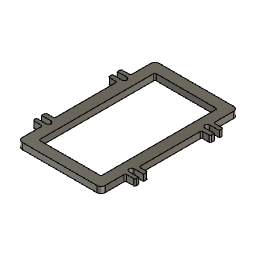
Model 2 v1 (Autodesk Fusion 360 design; units mm, degrees)
Autodesk Fusion 360 part; units mm, degrees
sketch "Sketch1" plane through (0, 0, 0) normal (0, 0, 1) x (1, 0, 0)
  line L0 (242.5602, 1007.653) -> (332.5602, 1007.653)
  line L1 (232.5602, 997.653) -> (232.5602, 952)
  line L2 (229.5602, 949) -> (212.5602, 949)
  line L3 (209.5602, 946) -> (209.5602, 940)
  line L4 (209.5602, 940) -> (229.5602, 940)
  arc A0 (242.5602, 1007.653) -> (232.5602, 997.653) centre (242.5602, 997.653) ccw
  line L5 (260.5602, 982.653) -> (332.5602, 982.653)
  line L6 (229.5602, 928) -> (209.5602, 928)
  line L7 (209.5602, 928) -> (209.5602, 921.1082)
  line L8 (212.5602, 918.1082) -> (227.6643, 918.1082)
  line L9 (229.5602, 940) -> (232.5602, 940)
  line L10 (229.5602, 928) -> (232.5602, 928)
  arc A1 (232.5602, 928) -> (232.5602, 940) centre (232.5602, 934) ccw
  line L11 (230.6643, 915.1082) -> (230.6643, 842.653)
  line L12 (257.5602, 979.653) -> (257.5602, 842.653)
  arc A2 (229.5602, 949) -> (232.5602, 952) centre (229.5602, 952) ccw
  arc A3 (230.6643, 915.1082) -> (227.6643, 918.1082) centre (227.6643, 915.1082) ccw
  arc A4 (212.5602, 949) -> (209.5602, 946) centre (212.5602, 946) ccw
  arc A5 (209.5602, 921.1082) -> (212.5602, 918.1082) centre (212.5602, 921.1082) ccw
  line L13 (435.5602, 949) -> (452.5602, 949)
  arc A6 (432.5602, 940) -> (432.5602, 928) centre (432.5602, 934) ccw
  line L14 (435.5602, 928) -> (432.5602, 928)
  line L15 (407.5602, 979.653) -> (407.5602, 842.653)
  line L16 (434.4561, 915.1082) -> (434.4561, 842.653)
  arc A7 (432.5602, 952) -> (435.5602, 949) centre (435.5602, 952) ccw
  line L17 (452.5602, 918.1082) -> (437.4561, 918.1082)
  arc A8 (432.5602, 997.653) -> (422.5602, 1007.653) centre (422.5602, 997.653) ccw
  line L18 (435.5602, 940) -> (432.5602, 940)
  arc A9 (437.4561, 918.1082) -> (434.4561, 915.1082) centre (437.4561, 915.1082) ccw
  arc A10 (452.5602, 918.1082) -> (455.5602, 921.1082) centre (452.5602, 921.1082) ccw
  line L19 (455.5602, 940) -> (435.5602, 940)
  line L20 (455.5602, 946) -> (455.5602, 940)
  line L21 (455.5602, 928) -> (455.5602, 921.1082)
  line L22 (422.5602, 1007.653) -> (332.5602, 1007.653)
  line L23 (404.5602, 982.653) -> (332.5602, 982.653)
  line L24 (432.5602, 997.653) -> (432.5602, 952)
  line L25 (435.5602, 928) -> (455.5602, 928)
  arc A11 (455.5602, 946) -> (452.5602, 949) centre (452.5602, 946) ccw
  line L26 (435.5602, 757.3059) -> (432.5602, 757.3059)
  line L27 (232.5602, 687.653) -> (232.5602, 733.3059)
  arc A12 (227.6643, 767.1978) -> (230.6643, 770.1978) centre (227.6643, 770.1978) ccw
  arc A13 (435.5602, 736.3059) -> (432.5602, 733.3059) centre (435.5602, 733.3059) ccw
  line L28 (212.5602, 767.1978) -> (227.6643, 767.1978)
  line L29 (455.5602, 757.3059) -> (455.5602, 764.1978)
  line L30 (229.5602, 757.3059) -> (232.5602, 757.3059)
  line L31 (435.5602, 736.3059) -> (452.5602, 736.3059)
  arc A14 (422.5602, 677.653) -> (432.5602, 687.653) centre (422.5602, 687.653) ccw
  line L32 (209.5602, 745.3059) -> (229.5602, 745.3059)
  arc A15 (209.5602, 739.3059) -> (212.5602, 736.3059) centre (212.5602, 739.3059) ccw
  arc A16 (232.5602, 733.3059) -> (229.5602, 736.3059) centre (229.5602, 733.3059) ccw
  arc A17 (232.5602, 687.653) -> (242.5602, 677.653) centre (242.5602, 687.653) ccw
  line L33 (455.5602, 739.3059) -> (455.5602, 745.3059)
  arc A18 (455.5602, 764.1978) -> (452.5602, 767.1978) centre (452.5602, 764.1978) ccw
  line L34 (209.5602, 757.3059) -> (209.5602, 764.1978)
  line L35 (229.5602, 745.3059) -> (232.5602, 745.3059)
  line L36 (209.5602, 739.3059) -> (209.5602, 745.3059)
  arc A19 (432.5602, 757.3059) -> (432.5602, 745.3059) centre (432.5602, 751.3059) ccw
  line L37 (455.5602, 745.3059) -> (435.5602, 745.3059)
  arc A20 (434.4561, 770.1978) -> (437.4561, 767.1978) centre (437.4561, 770.1978) ccw
  line L38 (435.5602, 757.3059) -> (455.5602, 757.3059)
  line L39 (432.5602, 687.653) -> (432.5602, 733.3059)
  line L40 (452.5602, 767.1978) -> (437.4561, 767.1978)
  line L41 (435.5602, 745.3059) -> (432.5602, 745.3059)
  arc A21 (452.5602, 736.3059) -> (455.5602, 739.3059) centre (452.5602, 739.3059) ccw
  arc A22 (212.5602, 767.1978) -> (209.5602, 764.1978) centre (212.5602, 764.1978) ccw
  line L42 (229.5602, 736.3059) -> (212.5602, 736.3059)
  line L43 (260.5602, 702.653) -> (332.5602, 702.653)
  line L44 (404.5602, 702.653) -> (332.5602, 702.653)
  arc A23 (232.5602, 745.3059) -> (232.5602, 757.3059) centre (232.5602, 751.3059) ccw
  line L45 (242.5602, 677.653) -> (332.5602, 677.653)
  line L46 (422.5602, 677.653) -> (332.5602, 677.653)
  line L47 (229.5602, 757.3059) -> (209.5602, 757.3059)
  line L48 (230.6643, 842.653) -> (230.6643, 770.1978)
  line L49 (257.5602, 842.653) -> (257.5602, 705.653)
  line L50 (407.5602, 842.653) -> (407.5602, 705.653)
  line L51 (434.4561, 842.653) -> (434.4561, 770.1978)
  arc A24 (407.5602, 979.653) -> (404.5602, 982.653) centre (404.5602, 979.653) ccw
  arc A25 (404.5602, 702.653) -> (407.5602, 705.653) centre (404.5602, 705.653) ccw
  arc A26 (260.5602, 982.653) -> (257.5602, 979.653) centre (260.5602, 979.653) ccw
  arc A27 (257.5602, 705.653) -> (260.5602, 702.653) centre (260.5602, 705.653) ccw
  point P0 (750, 0)
  point P1 (232.5602, 1007.653)
  point P2 (432.5602, 1007.653)
  point P3 (232.5602, 677.653)
  point P4 (432.5602, 677.653)
  dimension "d18" = 10
  dimension "d28" = 25
  dimension "d59" = 3
  dimension "d60" = 3
  dimension "d61" = 3
  dimension "d62" = 3
  dimension "d63" = 3
  dimension "d64" = 3
  dimension "d65" = 3
  dimension "d66" = 3
  constraint horizontal L0
  constraint perpendicular L0 L1
  constraint perpendicular L1 L2
  constraint perpendicular L2 L3
  constraint perpendicular L3 L4
  constraint coincident P1 L0
  constraint coincident P1 L1
  constraint tangent L0 A0
  constraint tangent L1 A0
  constraint perpendicular L6 L7
  constraint perpendicular L7 L8
  constraint parallel L4 L9
  constraint perpendicular L3 L10
  constraint tangent L9 A1
  constraint tangent L10 A1
  constraint perpendicular L8 L11
  constraint perpendicular L5 L12
  constraint tangent L1 A2
  constraint tangent L2 A2
  constraint tangent L8 A3
  constraint tangent L11 A3
  constraint tangent L2 A4
  constraint tangent L3 A4
  constraint tangent L7 A5
  constraint tangent L8 A5
  constraint perpendicular L43 L49
  constraint tangent L15 A24
  constraint tangent L23 A24
  constraint tangent L44 A25
  constraint tangent L50 A25
  constraint tangent L5 A26
  constraint tangent L12 A26
  constraint tangent L43 A27
  constraint tangent L49 A27
  measures "d18" radius of A0
  measures "d28" distance of L0.end L5
  measures "d59" radius of A2
  measures "d60" radius of A3
  measures "d61" radius of A4
  measures "d62" radius of A5
  measures "d63" radius of A24
  measures "d64" radius of A25
  measures "d65" radius of A26
  measures "d66" radius of A27
extrude "Extrude1" add sketch "Sketch1" along normal blind 15
